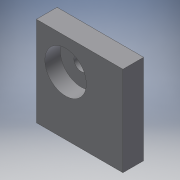
# Autodesk Inventor part: ZBaringBracket
Saved by Autodesk Inventor 2019 (Build 230136000, 136)
## iProperties
Created: 2018-10-14
Part Number: ZBaringBracket
Material: Generic
Document SubType Name: Modeling
Designer: LillaHunden
Density: 1 g/cm^3
Appearance: Default
Author: LillaHunden
Autodesk Inventor part; units mm, degrees
ref_plane "YZ Plane" through (0, 0, 0) normal (1, 0, 0) x (0, 1, 0)
ref_plane "XZ Plane" through (0, 0, 0) normal (0, 1, 0) x (-1, 0, 0)
ref_plane "XY Plane" through (0, 0, 0) normal (0, 0, 1) x (1, 0, 0)
sketch "Sketch1" plane through (0, 0, 0) normal (0, 0, 1) x (1, 0, 0)
  line L0 (6, -5.5) -> (6, -7.5) construction
  line L1 (6, -7.5) -> (25, -7.5) construction
  line L2 (25, -7.5) -> (25, 7.5) construction
  line L3 (25, 7.5) -> (7.55, 7.5) construction
  line L4 (7.55, 7.5) -> (7.55, 2.5) construction
  line L5 (7.55, 2.5) -> (-7.55, 2.5) construction
  line L6 (-7.55, 2.5) -> (-7.55, 7.5) construction
  line L7 (-7.55, 7.5) -> (-25, 7.5) construction
  line L8 (-25, 7.5) -> (-25, -7.5) construction
  line L9 (-25, -7.5) -> (-6, -7.5) construction
  line L10 (-6, -7.5) -> (-6, -5.5) construction
  line L11 (-6, -5.5) -> (6, -5.5) construction
  line L12 (-7.45, 15.5) -> (7.55, 15.5) construction
  line L13 (-7.45, 2.5) -> (-7.45, 15.5) construction
  line L14 (7.55, 2.5) -> (-7.45, 2.5) construction
  line L15 (7.55, 2.5) -> (7.55, 15.5) construction
  line L16 (25, -7.5) -> (-34.185, -7.5)
  line L17 (-34.185, -7.5) -> (-34.185, 35.7282)
  line L18 (-34.185, 35.7282) -> (25, 35.7282)
  line L19 (25, 35.7282) -> (25, -7.5)
  point P0 (0, 0)
  constraints: 8 end point, 2 parallel, 1 horizontal, 1 perpendicular, 1 point on line
extrude "Extrusion1" add sketch "Sketch1" along normal blind 10
sketch "Sketch2" plane through (0, 0, 10) normal (0, 0, 1) x (1, 0, 0)
  circle A0 centre (-20.1, 20.7) radius 2.5 construction
  circle A1 centre (-20.1, 20.7) radius 10
  point P0 (0, 0)
  dimension "BeringOD" = 20
  constraints: 1 centre point, 1 coincident
  measures "BeringOD" diameter of A1
extrude "Extrusion2" cut sketch "Sketch2" against normal blind 7.5
sketch "Sketch3" plane through (-20.1, 20.7, 2.5) normal (0, 0, 1) x (1, 0, 0)
  circle A0 centre (0, 0) radius 3.5
  point P0 (20.1, -20.7)
  dimension "BaringID" = 7
  constraints: 1 centre point
  measures "BaringID" diameter of A0
extrude "Extrusion3" cut sketch "Sketch3" against normal through all
body "Solid1"
